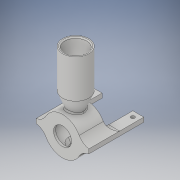
# Autodesk Inventor part: powderTurnRes
Saved by Autodesk Inventor 2017 (Build 210142000, 142)
## iProperties
Created: 2019-05-09
Part Number: powderTurnRes
Material: Generic
Document SubType Name: Modeling
Designer: Joe Sedutto
Density: 1 g/cm^3
Appearance: Default
Author: Joe Sedutto
Autodesk Inventor part; units mm, degrees
ref_plane "YZ Plane" through (0, 0, 0) normal (1, 0, 0) x (0, 1, 0)
sketch "Sketch1" plane through (0, 0, 0) normal (0, 0, 1) x (1, 0, 0)
  circle A0 centre (0, 0) radius 15.494
  circle A1 centre (0, 0) radius 21.844
  dimension "d0" = 30.988
  dimension "d1" = 6.35
  constraints: 2 centre point, 1 coincident
  measures "d0" diameter of A0
  measures "d1" radial gap between concentric circles of A0 A1
extrude "Extrusion1" add sketch "Sketch1" along normal blind 25.4
sketch "Sketch2" plane through (0, 0, 25.4) normal (0, 0, 1) x (1, 0, 0)
  circle A0 centre (0, 0) radius 15.494 projected
  circle A1 centre (0, 0) radius 21.844 projected
  circle A2 centre (0, 0) radius 10.414
  dimension "d4" = 5.08
  constraints: 1 centre point
  measures "d4" radial gap between concentric circles of A0 A2
extrude "Extrusion2" add sketch "Sketch2" along normal blind 2.54 contours A0 | A1
ref_plane "Work Plane1" through (0, 21.844, 0) normal (0, 1, 0) x (-1, 0, 0)
sketch "Sketch3" plane through (0, 21.844, 0) normal (0, 1, 0) x (-1, 0, 0)
  line L0 (-15.494, 0) -> (-15.494, 25.4) projected
  line L1 (0, 12.7) -> (-15.494, 12.7) construction
  line L2 (15.494, 0) -> (15.494, 25.4) projected
  line L3 (15.494, 12.7) -> (0, 12.7) construction
  point P0 (0, 0)
  constraints: 4 end point, 2 midpoint, 1 collinear, 1 horizontal
hole "Hole1" at (0, 21.844, 12.7) direction (0, -1, 0) diameter 8.89 depth 12.7 tip angle 118
ref_plane "Work Plane2" through (0, 0, 12.7) normal (0, 0, -1) x (-1, 0, 0)
sketch "Sketch4" plane through (0, 0, 12.7) normal (0, 0, -1) x (-1, 0, 0)
  line L0 (-4.445, 17.3827) -> (-12.7, 38.1)
  line L1 (-12.7, 38.1) -> (-15.24, 38.1)
  line L2 (-15.24, 38.1) -> (-6.985, 17.3827)
  line L3 (-6.985, 17.3827) -> (-4.445, 17.3827)
  circle A0 centre (0, 0) radius 21.844 projected
  line L4 (0, 21.844) -> (0, 32.8531) construction
  line L5 (-4.445, 14.8427) -> (-4.445, 21.387) projected
  line L6 (0, 21.844) -> (0, 0) construction
  dimension "d15" = 2.54
  dimension "d16" = 38.1
  dimension "d18" = 2.54
  dimension "d51" = 15.24
  constraints: 12 end point, 2 parallel, 1 collinear, 1 horizontal, 1 point on circle, 1 point on line, 1 vertical
  measures "d15" distance of L0.end L1.end
  measures "d16" distance from line of L1 point (0, 0)
  measures "d18" distance of L0.start L5.start
  measures "d51" distance from line of L4 L1.end
revolve "Revolution1" add sketch "Sketch4" angle 360 about axis through (0, 21.844, 12.7) along (0, 1, 0) contours L3 L2 A0 L0 | A0 L2 L1 L0
sketch "Sketch5" plane through (0, 38.1, 12.7) normal (0, 1, 0) x (1, 0, 0)
  circle A0 centre (0, 0) radius 15.24 projected
  circle A1 centre (0, 0) radius 12.7 projected
  point P0 (0, 12.7)
extrude "Extrusion3" add sketch "Sketch5" along normal blind 44.45
fillet "Fillet1" radius 1.27 1 edges at (-12.7, 82.55, 12.7)
fillet "Fillet2" radius 1.27 1 edges at (-8.1363, 20.2722, 12.6995)
sketch "Sketch7" plane through (0, 0, 0) normal (0, 1, 0) x (-1, 0, 0)
  spline S0 degree 5 poles (0, 17.145) (0.4828, 17.145) (0.9596, 17.0794) (1.4131, 16.9518) (1.8298, 16.7732) (2.5558, 16.3598) (2.8734, 16.1246) (3.1532, 15.8657) (3.3965, 15.5895) (3.9479, 14.8249) (4.1981, 14.3133) (4.3627, 13.7816) (4.445, 13.2414) (4.445, 11.8392) (4.2363, 10.9863) (3.8286, 10.1691) (3.1783, 9.4173) (1.6788, 8.5276) (0.9446, 8.2456) (0.1197, 8.1438) (-0.6891, 8.2446) (-2.2793, 8.7739) (-2.9916, 9.2632) (-3.5287, 9.8467) (-3.9168, 10.482) (-4.4234, 11.8402) (-4.5299, 12.5666) (-4.4933, 13.2974) (-4.312, 14.0161) (-3.8386, 14.9618) (-3.677, 15.2265) (-3.4889, 15.4821) (-3.2733, 15.7257) (-2.77, 16.1943) (-2.4777, 16.4184) (-2.1517, 16.6188) (-1.7928, 16.788) (-1.1419, 17.0047) (-0.8666, 17.0738) (-0.5815, 17.1212) (-0.2911, 17.145) (0, 17.145) knots 0 0 0 0 0 0 0.07101 0.07101 0.07101 0.07101 0.139421 0.139421 0.139421 0.139421 0.251612 0.251612 0.251612 0.251612 0.429979 0.429979 0.429979 0.429979 0.545472 0.545472 0.545472 0.545472 0.686985 0.686985 0.686985 0.686985 0.834646 0.834646 0.834646 0.834646 0.894296 0.894296 0.894296 0.894296 0.957486 0.957486 0.957486 0.957486 1 1 1 1 1 1
  spline S1 degree 5 poles (0, 18.415) (1.4735, 18.4148) (2.948, 17.941) (4.2156, 16.9874) (5.8346, 14.5842) (5.8574, 11.7206) (5.4821, 10.4159) (3.8546, 7.8689) (0.9939, 6.7002) (-0.7875, 6.6697) (-3.7108, 7.7484) (-5.429, 10.2708) (-5.8437, 11.5935) (-5.8728, 14.5019) (-4.2541, 16.9581) (-2.978, 17.9314) (-1.4885, 18.4147) (0, 18.415) knots 0 0 0 0 0 0 0.205202 0.205202 0.205202 0.383994 0.383994 0.383994 0.610546 0.610546 0.610546 0.792713 0.792713 0.792713 1 1 1 1 1 1
  point P0 (0, 0)
  dimension "d30" = 1.27
  constraints: 3 other
extrude "Extrusion5" cut sketch "Sketch7" against normal blind 25.4 contours S0 | S1
chamfer "Chamfer2" distance 3.175 angle 45 1 edges at (0, -15.494, 6.9851)
sketch "Sketch8" plane through (0, 0, 0) normal (0, 1, 0) x (-1, 0, 0)
  line L0 (21.844, 27.94) -> (-21.844, 27.94) projected
  line L1 (17.78, 27.94) -> (30.48, 27.94)
  line L2 (30.48, 27.94) -> (30.48, -35.56)
  line L3 (30.48, -35.56) -> (17.78, -35.56)
  line L4 (17.78, -35.56) -> (17.78, 27.94)
  line L5 (0, 27.94) -> (0, -2.54) construction
  circle A0 centre (0, 12.7) radius 15.24 projected
  line L6 (-21.844, 27.94) -> (21.844, 27.94)
  line L7 (-17.78, 27.94) -> (-30.48, 27.94)
  line L8 (-30.48, 27.94) -> (-30.48, -35.56)
  line L9 (-30.48, -35.56) -> (-17.78, -35.56)
  line L10 (-17.78, -35.56) -> (-17.78, 27.94)
  circle A1 centre (0, 12.7) radius 15.24
  point P0 (0, 0)
  dimension "d36" = 12.7
  dimension "d37" = 17.78
  dimension "d38" = 63.5
  constraints: 20 end point, 6 symmetric about line, 2 parallel, 2 point on line, 1 centre point, 1 horizontal, 1 line through centre, 1 midpoint, 1 perpendicular, 1 vertical, 1 vertical alignment, 1 other
  measures "d36" distance between parallel lines of L4 L2
  measures "d37" distance from line of A1.centre L4
  measures "d38" distance between parallel lines of L1 L3
extrude "Extrusion6" add sketch "Sketch8" along normal mid plane 5.08 contours L1 L2 L3 L4 L0 | L10 L9 L8 L7 L0
fillet "Fillet3" radius 15.24 4 edges at (21.6958, 2.54, 13.97) (-21.6958, 2.54, 13.97) (-21.6958, -2.54, 13.97) (21.6958, -2.54, 13.97)
sketch "Sketch9" plane through (0, 2.54, 0) normal (0, 1, 0) x (1, 0, 0)
  line L0 (17.78, 35.56) -> (17.78, 0) projected
  line L1 (30.48, 35.56) -> (17.78, 35.56)
  line L2 (17.78, 35.56) -> (17.78, 22.86)
  line L3 (17.78, 22.86) -> (30.48, 22.86)
  line L4 (30.48, 22.86) -> (30.48, 35.56)
  line L5 (30.48, 35.56) -> (17.78, 22.86) construction
  line L6 (17.78, 35.56) -> (30.48, 22.86) construction
  line L7 (-30.48, 0) -> (-30.48, 35.56) projected
  line L8 (-17.78, 35.56) -> (-30.48, 35.56)
  line L9 (-30.48, 35.56) -> (-30.48, 22.86)
  line L10 (-30.48, 22.86) -> (-17.78, 22.86)
  line L11 (-17.78, 22.86) -> (-17.78, 35.56)
  line L12 (-17.78, 35.56) -> (-30.48, 22.86) construction
  line L13 (-30.48, 35.56) -> (-17.78, 22.86) construction
  line L14 (30.48, 35.56) -> (17.78, 35.56) projected
  line L15 (30.48, 0) -> (30.48, 35.56) projected
  line L16 (-17.78, 35.56) -> (-30.48, 35.56) projected
  line L17 (-17.78, 0) -> (-17.78, 35.56) projected
  point P0 (0, 0)
  point P1 (24.13, 29.21)
  point P2 (-30.48, -27.94)
  point P3 (-24.13, 29.21)
  point P4 (30.48, -27.94)
  point P5 (24.13, 29.21)
  point P6 (-24.13, 29.21)
  constraints: 24 end point, 4 collinear, 4 midpoint, 4 parallel, 3 perpendicular, 3 point on line, 2 coincident, 2 horizontal
hole "Hole2" at (24.13, 2.54, -29.21) at (-24.13, 2.54, -29.21) direction (0, -1, 0) diameter 4.2333 depth 12.7 tip angle 118
fillet "Fillet4" radius 7.62 4 edges at (-24.13, 2.54, 0) (24.13, 2.54, 0) (-24.13, -2.54, 0) (24.13, -2.54, 0)
fillet "Fillet5" radius 1.27 2 edges at (-17.78, 0, 0) (17.78, 0, 0)
body "Solid1"
